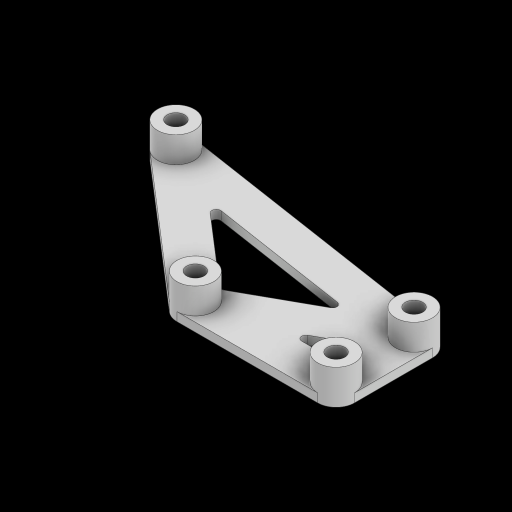
# Autodesk Inventor part: 200_Frame_Internal
Saved by Autodesk Inventor 2024 (Build 280153000, 153)
## iProperties
Created: 2023-07-20
Part Number: 200_Frame_Internal
Material: Generisch
Document SubType Name: Modeling
Designer: Philipp
Density: 1 g/cm^3
Appearance: Vorgabe
Author: Philipp
Autodesk Inventor part; units mm, degrees
ref_plane "YZ Plane" through (0, 0, 0) normal (1, 0, 0) x (0, 1, 0)
ref_plane "XZ Plane" through (0, 0, 0) normal (0, 1, 0) x (-1, 0, 0)
ref_plane "XY Plane" through (0, 0, 0) normal (0, 0, 1) x (1, 0, 0)
sketch "Skizze1" plane through (0, 0, 0) normal (0, 0, 1) x (1, 0, 0)
  circle A0 centre (5, 33) radius 4.25
  circle A1 centre (37.5, 5) radius 4.25
  circle A2 centre (70, 23) radius 4.25
  circle A3 centre (70, 5) radius 4.25
  circle A4 centre (5, 33) radius 2
  circle A5 centre (37.5, 5) radius 2
  circle A6 centre (70, 5) radius 2
  circle A7 centre (70, 23) radius 2
  point P0 (0, 0)
  dimension "d0" = 8.5
  dimension "d1" = 33
  dimension "d2" = 5
  dimension "d3" = 8.5
  dimension "d4" = 5
  dimension "d5" = 37.5
  dimension "d6" = 8.5
  dimension "d7" = 70
  dimension "d8" = 23
  dimension "d9" = 8.5
  dimension "d10" = 70
  dimension "d11" = 5
  dimension "d12" = 4
  dimension "d13" = 4
  dimension "d14" = 4
  dimension "d15" = 4
  constraints: 8 centre point, 4 coincident
  measures "d0" diameter of A0
  measures "d1" vertical distance of point (0, 0) A0.centre
  measures "d2" horizontal distance of point (0, 0) A0.centre
  measures "d3" diameter of A1
  measures "d4" vertical distance of point (0, 0) A1.centre
  measures "d5" horizontal distance of point (0, 0) A1.centre
  measures "d6" diameter of A2
  measures "d7" horizontal distance of point (0, 0) A2.centre
  measures "d8" vertical distance of point (0, 0) A2.centre
  measures "d9" diameter of A3
  measures "d10" horizontal distance of point (0, 0) A3.centre
  measures "d11" vertical distance of point (0, 0) A3.centre
  measures "d12" diameter of A4
  measures "d13" diameter of A5
  measures "d14" diameter of A6
  measures "d15" diameter of A7
extrude "Extrusion1" add sketch "Skizze1" against normal blind 8
sketch "Skizze2" plane through (70, 23, -8) normal (0, 0, -1) x (-1, 0, 0)
  circle A0 centre (0, 0) radius 2 projected
  circle A1 centre (0, 0) radius 4.25 projected
  circle A2 centre (0, 0) radius 2 projected
  circle A3 centre (0, -18) radius 4.25 projected
  circle A4 centre (0, -18) radius 2 projected
  circle A5 centre (32.5, -18) radius 4.25 projected
  circle A6 centre (32.5, -18) radius 2 projected
  circle A7 centre (65, 10) radius 4.25 projected
  circle A8 centre (65, 10) radius 2 projected
  line L0 (0, 0) -> (0, -18) construction
  line L1 (-4.25, 0) -> (-4.25, -18)
  line L2 (4.25, -18) -> (4.25, 0)
  arc A9 (4.25, 0) -> (-4.25, 0) centre (0, 0) ccw
  arc A10 (-4.25, -18) -> (4.25, -18) centre (0, -18) ccw
  line L3 (0, -18) -> (32.5, -18) construction
  line L4 (0, -22.25) -> (32.5, -22.25)
  line L5 (32.5, -13.75) -> (0, -13.75)
  arc A11 (0, -13.75) -> (0, -22.25) centre (0, -18) ccw
  arc A12 (32.5, -22.25) -> (32.5, -13.75) centre (32.5, -18) ccw
  circle A13 centre (32.5, -18) radius 2 projected
  line L6 (65, 10) -> (32.5, -18) construction
  line L7 (62.226, 13.2198) -> (29.726, -14.7802)
  line L8 (35.274, -21.2198) -> (67.774, 6.7802)
  arc A14 (67.774, 6.7802) -> (62.226, 13.2198) centre (65, 10) ccw
  arc A15 (29.726, -14.7802) -> (35.274, -21.2198) centre (32.5, -18) ccw
  line L9 (0, 0) -> (32.5, -18) construction
  line L10 (-2.0591, -3.7179) -> (30.4409, -21.7179)
  line L11 (34.5591, -14.2821) -> (2.0591, 3.7179)
  arc A16 (2.0591, 3.7179) -> (-2.0591, -3.7179) centre (0, 0) ccw
  arc A17 (30.4409, -21.7179) -> (34.5591, -14.2821) centre (32.5, -18) ccw
  line L12 (0, 0) -> (65, 10) construction
  line L13 (0.6462, -4.2006) -> (65.6462, 5.7994)
  line L14 (64.3538, 14.2006) -> (-0.6462, 4.2006)
  arc A18 (-0.6462, 4.2006) -> (0.6462, -4.2006) centre (0, 0) ccw
  arc A19 (65.6462, 5.7994) -> (64.3538, 14.2006) centre (65, 10) ccw
  point P0 (70, -23)
  point P1 (0, -9)
  point P2 (16.25, -18)
  point P3 (48.75, -4)
  point P4 (16.25, -9)
  point P5 (32.5, 5)
  point P6 (50.9971, 3.5457)
  point P7 (31.9691, -12.8477)
  point P8 (12.9411, -2.3091)
  point P9 (-4.25, 0)
  point P10 (-4.25, -18)
  point P11 (4.25, -13.75)
  point P12 (4.25, -7.2121)
  point P13 (16.0545, -13.75)
  constraints: 40 end point, 20 point on circle, 20 tangent, 10 centre point, 5 midpoint, 5 parallel, 4 concentric, 1 perpendicular, 1 vertical
extrude "Extrusion2" add sketch "Skizze2" against normal blind 2 contours A0 | L2 L13 A1 | A1 L11 L13 L2 | A1 L14 A7 L7 L13 L11 | L13 L2 L10 A1 | L13 L11 L7 L5 L10 L2 | L10 L2 L5 A3 L1 A1 | L11 A5 L5 L7 | L7 L13 A7 L8 A5 L11 | L7 A7 L13 | L5 L10 A5 L4 A3 L2 | L2 A3 L5 | L5 L7 A5 L10 | L5 A5 L7 | A4 | A6 | A8
fillet "Rundung1" radius 1 6 edges at (19.0029, 26.5457, -7) (38.0309, 10.1523, -7) (57.0589, 20.6909, -7) (53.9455, 9.25, -7) (65.75, 9.25, -7) (65.75, 15.7879, -7)
